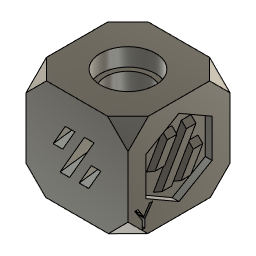
Voron_Design_Cube_v7 (Autodesk Fusion 360 design; units mm, degrees)
Autodesk Fusion 360 part; units mm, degrees
note: some values were not read from the file. Chosen so that the rebuilt part matches the saved one: which bodies a step acts on; the sign of a taper; which pieces of a blend or face edit are solid.
sketch "Sketch1" plane through (0, 0, 0) normal (1, 0, 0) x (0, 1, 0) in component "Voron_Design_Cube_v7"
  line L0 (15, -15) -> (-15, -15)
  line L1 (-15, -15) -> (-15, 15)
  line L2 (-15, 15) -> (15, 15)
  line L3 (15, 15) -> (15, -15)
  line L4 (15, -15) -> (-15, 15) construction
  line L5 (-15, -15) -> (15, 15) construction
  dimension "d4" = 30
  dimension "d5" = 30
  constraint horizontal L0
  constraint perpendicular L0 L1
  constraint parallel L0 L2
  constraint parallel L1 L3
  constraint coincident L4 origin
  constraint coincident L5 origin
  measures "d4" distance of L1.end L2.end
  measures "d5" distance of L0.end L1.end
extrude "Extrude1" add sketch "Sketch1" along normal mid plane 30 makes body 1 in component "Voron_Design_Cube_v7"
sketch "Sketch2" plane through (0, 0, 15) normal (0, 0, 1) x (-1, 0, 0) in component "Voron_Design_Cube_v7"
  line L0 (15, 15) -> (-15, 15)
  line L1 (-15, 15) -> (-15, -15)
  line L2 (-15, -15) -> (15, -15)
  line L3 (15, -15) -> (15, 15)
  circle A0 centre (0, 0) radius 8.1
  circle A1 centre (0, 0) radius 6.6
  dimension "d6" = 16.2
  dimension "d7" = 13.2
  constraint coincident A0.centre A1.centre
  measures "d6" diameter of A0
  measures "d7" diameter of A1
extrude "Extrude2" cut sketch "Sketch2" against normal through all contours A1 picked at (1.732843, 1.802463) bodies 1 in component "Voron_Design_Cube_v7"
extrude "Extrude3" cut sketch "Sketch2" against normal blind 5.2 contours A0 picked at (7.545271, -0.730307) bodies 1 in component "Voron_Design_Cube_v7"
sketch "Sketch3" plane through (0, 0, -15) normal (0, 0, -1) x (1, 0, 0) in component "Voron_Design_Cube_v7"
  circle A0 centre (0, 0) radius 6.6
  line L0 (-15, -15) -> (15, -15)
  line L1 (15, -15) -> (15, 15)
  line L2 (15, 15) -> (-15, 15)
  line L3 (-15, 15) -> (-15, -15)
  circle A1 centre (0, 0) radius 7.65
  dimension "d11" = 15.3
  constraint coincident A0.centre A1.centre
  measures "d11" diameter of A1
extrude "Extrude4" cut sketch "Sketch3" against normal blind 1.2 contours A0 | A1 picked at (1.732843, 1.802463) picked at (7.246947, -0.707951) bodies 1 in component "Voron_Design_Cube_v7"
sketch "Sketch4" plane through (0, 0, -13.8) normal (0, 0, -1) x (1, 0, 0) in component "Voron_Design_Cube_v7"
  circle A0 centre (0, 0) radius 6.6
  circle A1 centre (0, 0) radius 7.65
  circle A2 centre (0, 0) radius 7.625
  dimension "d14" = 15.25
  constraint concentric A0 A2
  measures "d14" diameter of A2
extrude "Extrude5" cut sketch "Sketch4" against normal through all draft -45 contours A0 | A1 A2 picked at (1.732843, 1.802463) picked at (7.246947, -0.707951) bodies 1 in component "Voron_Design_Cube_v7"
sketch "Sketch6" plane through (0, 0, 15) normal (0, 0, 1) x (-1, 0, 0) in component "Voron_Design_Cube_v7"
  circle A0 centre (0, 0) radius 8.1
  line L0 (15, 15) -> (-15, 15)
  line L1 (-15, 15) -> (-15, -15)
  line L2 (-15, -15) -> (15, -15)
  line L3 (15, -15) -> (15, 15)
  point P0 (9, -15)
  point P1 (15, -9)
  point P2 (15, 9)
  point P3 (9, 15)
  point P4 (-9, 15)
  point P5 (-15, 9)
  point P6 (-15, -9)
  point P7 (-9, -15)
  dimension "d20" = 6
  dimension "d21" = 6
  dimension "d23" = 360
  constraint coincident L2 P0
  constraint coincident L3 P1
  measures "d20" distance of L2.end P0
  measures "d21" distance of L2.end P1
sketch "Sketch7" plane through (0, 0, -15) normal (0, 0, -1) x (1, 0, 0) in component "Voron_Design_Cube_v7"
  circle A0 centre (0, 0) radius 7.65
  line L0 (-15, -15) -> (15, -15)
  line L1 (15, -15) -> (15, 15)
  line L2 (15, 15) -> (-15, 15)
  line L3 (-15, 15) -> (-15, -15)
  point P0 (-15, 9.040867)
  point P1 (-9, 15)
  point P2 (-15, -9)
  point P3 (-9.040867, -15)
  point P4 (9, -15)
  point P5 (15, -9.040867)
  point P6 (15, 9)
  point P7 (9.040867, 15)
  dimension "d25" = 360
  constraint coincident L2 P1
sketch "Sketch8" plane through (15, 0, 0) normal (1, 0, 0) x (0, 1, 0) in component "Voron_Design_Cube_v7"
  line L0 (15, 15) -> (-15, 15)
  line L1 (-15, 15) -> (-15, -15)
  line L2 (-15, -15) -> (15, -15)
  line L3 (15, -15) -> (15, 15)
  line L4 (0, 0) -> (0, 20) construction
  line L5 (0, 20) -> (0, 0) construction
  line L6 (0, 0) -> (20, 0) construction
  point P0 (-15, 9)
  point P1 (-15, 15)
  point P2 (15, 9)
  point P3 (-15, -9)
  point P4 (15, -9)
  dimension "d26" = 6
  constraint coincident L1 P0
  constraint coincident L4.start L5.end
  constraint vertical L4
  constraint parallel L4 L5
  constraint symmetric P0 L5 P2
  constraint perpendicular L5 L6
  constraint symmetric P0 L6 P3
  constraint symmetric P2 L6 P4
  measures "d26" distance of P0 P1
sketch "Sketch9" plane through (-15, 0, 0) normal (-1, 0, 0) x (0, -1, 0) in component "Voron_Design_Cube_v7"
  line L0 (15, 15) -> (-15, 15)
  line L1 (-15, 15) -> (-15, -15)
  line L2 (-15, -15) -> (15, -15)
  line L3 (15, -15) -> (15, 15)
  point P0 (-15, 9)
  point P1 (15, 9)
  point P2 (15, -9)
  point P3 (-15, -9)
ref_plane "WorkPlane1" through (-15, -9, 15) normal (0.57735, 0.57735, -0.57735) x (-0.707107, 0.707107, 0) in component "Voron_Design_Cube_v7"
ref_plane "WorkPlane2" through (9, -15, 15) normal (-0.57735, 0.57735, -0.57735) x (-0.707107, -0.707107, 0) in component "Voron_Design_Cube_v7"
ref_plane "WorkPlane3" through (15, 9, 15) normal (-0.57735, -0.57735, -0.57735) x (0.707107, -0.707107, 0) in component "Voron_Design_Cube_v7"
ref_plane "WorkPlane4" through (-9, 15, 15) normal (0.57735, -0.57735, -0.57735) x (0.707107, 0.707107, 0) in component "Voron_Design_Cube_v7"
ref_plane "WorkPlane5" through (-9.040867, 15, -15) normal (0.579981, -0.576031, 0.576031) x (0.704686, 0.709519, 0) in component "Voron_Design_Cube_v7"
ref_plane "WorkPlane6" through (-15, -9.040867, -15) normal (0.576031, 0.579981, 0.576031) x (-0.709519, 0.704686, 0) in component "Voron_Design_Cube_v7"
ref_plane "WorkPlane7" through (9.040867, -15, -15) normal (-0.579981, 0.576031, 0.576031) x (-0.704686, -0.709519, 0) in component "Voron_Design_Cube_v7"
ref_plane "WorkPlane8" through (15, 9.040867, -15) normal (-0.576031, -0.579981, 0.576031) x (0.709519, -0.704686, 0) in component "Voron_Design_Cube_v7"
split "Split1" by plane through (9, -15, 15) normal (-0.57735, 0.57735, -0.57735) bodies 1 makes body 2 at (6.567203, -0.657148, -5.25) in component "Voron_Design_Cube_v7"
delete_body "RemoveBody1" bodies 1 in component "Voron_Design_Cube_v7"
split "Split2" by plane through (15, 9, 15) normal (-0.57735, -0.57735, -0.57735) bodies 2 makes body 3 at (6.567203, -0.657148, -5.25) in component "Voron_Design_Cube_v7"
delete_body "RemoveBody2" bodies 2 in component "Voron_Design_Cube_v7"
split "Split3" by plane through (-9, 15, 15) normal (0.57735, -0.57735, -0.57735) bodies 3 makes body 4 at (6.567203, -0.657148, -5.25) in component "Voron_Design_Cube_v7"
delete_body "RemoveBody3" bodies 3 in component "Voron_Design_Cube_v7"
split "Split4" by plane through (-15, -9, 15) normal (0.57735, 0.57735, -0.57735) bodies 4 makes body 5 at (6.567203, -0.657148, -5.25) in component "Voron_Design_Cube_v7"
delete_body "RemoveBody4" bodies 4 in component "Voron_Design_Cube_v7"
split "Split5" by plane through (-15, -9.040867, -15) normal (0.576031, 0.579981, 0.576031) bodies 5 makes body 6 at (6.567203, -0.657148, -5.25) in component "Voron_Design_Cube_v7"
delete_body "RemoveBody5" bodies 5 in component "Voron_Design_Cube_v7"
split "Split6" by plane through (9.040867, -15, -15) normal (-0.579981, 0.576031, 0.576031) bodies 6 makes body 7 at (6.567203, -0.657148, -5.25) in component "Voron_Design_Cube_v7"
delete_body "RemoveBody6" bodies 6 in component "Voron_Design_Cube_v7"
split "Split7" by plane through (15, 9.040867, -15) normal (-0.576031, -0.579981, 0.576031) bodies 7 makes body 8 at (6.567203, -0.657148, -5.25) in component "Voron_Design_Cube_v7"
delete_body "RemoveBody7" bodies 7 in component "Voron_Design_Cube_v7"
split "Split8" by plane through (-9.040867, 15, -15) normal (0.579981, -0.576031, 0.576031) bodies 8 makes body 9 at (6.567203, -0.657148, -5.25) in component "Voron_Design_Cube_v7"
delete_body "RemoveBody8" bodies 8 in component "Voron_Design_Cube_v7"
sketch "Sketch10" plane through (0, 15, 0) normal (0, 1, 0) x (-1, 0, 0) in component "Voron_Design_Cube_v7"
  line L0 (9.040866, -15) -> (15, -9)
  line L1 (15, -9) -> (15, 9)
  line L2 (15, 9) -> (9, 15)
  line L3 (9, 15) -> (-9, 15)
  line L4 (-9, 15) -> (-15, 9)
  line L5 (-15, 9) -> (-15, -9)
  line L6 (-15, -9) -> (-9, -15)
  line L7 (-9, -15) -> (9.040866, -15)
  line L8 (-13, -13) -> (-7.5, -13) construction
  line L9 (-7.5, -13) -> (-7.5, -7) construction
  line L10 (-7.5, -7) -> (-13, -7) construction
  line L11 (-13, -7) -> (-13, -13) construction
  dimension "d27" = 5.7
  dimension "d30" = 13
  dimension "d31" = 13
  text T0 "X" font "Arial" height 5.7 align left bottom in box 5.5 x 6 at (-13, -13) x (1, 0) y (0, 1) spacing 1
  measures "d30" distance of origin
  measures "d31" distance of origin
extrude "Extrude6" cut sketch "Sketch10" against normal blind 2 text T0 bodies 9 in component "Voron_Design_Cube_v7"
sketch "Sketch11" plane through (15, 0, 0) normal (1, 0, 0) x (0, 1, 0) in component "Voron_Design_Cube_v7"
  line L0 (9.040867, -15) -> (15, -9)
  line L1 (15, -9) -> (15, 9)
  line L2 (15, 9) -> (9, 15)
  line L3 (9, 15) -> (-9, 15)
  line L4 (-9, 15) -> (-15, 9)
  line L5 (-15, 9) -> (-15, -9)
  line L6 (-15, -9) -> (-9, -15)
  line L7 (-9, -15) -> (9.040867, -15)
  line L8 (-13, -13) -> (-5.617602, -13) construction
  line L9 (-5.617602, -13) -> (-5.617602, -5.858994) construction
  line L10 (-5.617602, -5.858994) -> (-13, -5.858994) construction
  line L11 (-13, -5.858994) -> (-13, -13) construction
  dimension "d32" = 5.7
  dimension "d33" = 13
  dimension "d34" = 13
  text T0 "Y" font "Arial" height 5.7 align left bottom in box 7.382398 x 7.141006 at (-13, -13) x (1, 0) y (0, 1) spacing 1
  constraint horizontal L8
  measures "d33" distance of origin
  measures "d34" distance of origin
extrude "Extrude7" cut sketch "Sketch11" against normal blind 2 text T0 bodies 9 in component "Voron_Design_Cube_v7"
sketch "Sketch12" plane through (15, 0, 0) normal (1, 0, 0) x (0, 1, 0) in component "Voron_Design_Cube_v7"
  line L0 (-9.73799, 5.622396) -> (0, 11.244792)
  line L1 (0, 11.244792) -> (9.73799, 5.622396)
  line L2 (9.73799, 5.622396) -> (9.73799, -5.622396)
  line L3 (9.73799, -5.622396) -> (0, -11.244792)
  line L4 (0, -11.244792) -> (-9.73799, -5.622396)
  line L5 (-9.73799, -5.622396) -> (-9.73799, 5.622396)
  line L6 (-7.01675, 0) -> (-3.440906, 6.207125)
  line L7 (-3.440906, 6.207125) -> (-0.629708, 6.207125)
  line L8 (-0.629708, 6.207125) -> (-4.205552, 0)
  line L9 (-4.205552, 0) -> (-7.01675, 0)
  line L10 (2.18149, 6.207125) -> (4.992688, 6.207125)
  line L11 (4.992688, 6.207125) -> (-2.18149, -6.207125)
  line L12 (-2.18149, -6.207125) -> (-4.992688, -6.207125)
  line L13 (-4.992688, -6.207125) -> (2.18149, 6.207125)
  line L14 (4.205552, 0) -> (7.01675, 0)
  line L15 (7.01675, 0) -> (3.440906, -6.207125)
  line L16 (3.440906, -6.207125) -> (0.629708, -6.207125)
  line L17 (0.629708, -6.207125) -> (4.205552, 0)
extrude "Extrude8" cut sketch "Sketch12" against normal blind 2 bodies 9 in component "Voron_Design_Cube_v7"
draft "Draft1" angle 25 neutral plane through (15, 0, 0) pull (1, 0, 0) 6 faces at (14.333333, -2.50384, 6.207125) (14.333333, 3.118556, 6.207125) (14.333333, 5.142618, 0) (14.333333, -3.118556, -6.207125) (14.333333, 2.50384, -6.207125) (14.333333, -5.142618, 0) on bodies 9 in component "Voron_Design_Cube_v7"
sketch "Sketch13" plane through (-15, 0, 0) normal (-1, 0, 0) x (0, -1, 0) in component "Voron_Design_Cube_v7"
  line L0 (-15, -9) -> (-9, -15)
  line L1 (-9, -15) -> (9.040867, -15)
  line L2 (9.040867, -15) -> (15, -9)
  line L3 (15, -9) -> (15, 9)
  line L4 (15, 9) -> (9, 15)
  line L5 (9, 15) -> (-9, 15)
  line L6 (-9, 15) -> (-15, 9)
  line L7 (-15, 9) -> (-15, -9)
  line L8 (-9.73799, 5.622396) -> (0, 11.244792)
  line L9 (0, 11.244792) -> (9.73799, 5.622396)
  line L10 (9.73799, 5.622396) -> (9.73799, -5.622396)
  line L11 (9.73799, -5.622396) -> (0, -11.244792)
  line L12 (0, -11.244792) -> (-9.73799, -5.622396)
  line L13 (-9.73799, -5.622396) -> (-9.73799, 5.622396)
  line L14 (-7.01675, 0) -> (-3.440906, 6.207125)
  line L15 (-3.440906, 6.207125) -> (-0.629708, 6.207125)
  line L16 (-0.629708, 6.207125) -> (-4.205552, 0)
  line L17 (-4.205552, 0) -> (-7.01675, 0)
  line L18 (2.18149, 6.207125) -> (4.992688, 6.207125)
  line L19 (4.992688, 6.207125) -> (-2.18149, -6.207125)
  line L20 (-2.18149, -6.207125) -> (-4.992688, -6.207125)
  line L21 (-4.992688, -6.207125) -> (2.18149, 6.207125)
  line L22 (4.205552, 0) -> (7.01675, 0)
  line L23 (7.01675, 0) -> (3.440906, -6.207125)
  line L24 (3.440906, -6.207125) -> (0.629708, -6.207125)
  line L25 (0.629708, -6.207125) -> (4.205552, 0)
extrude "Extrude9" cut sketch "Sketch13" against normal blind 2 contours L8 L9 L10 L11 L12 L13 picked at (-6.731882, 3.943174) bodies 9 in component "Voron_Design_Cube_v7"
draft "Draft2" angle 25 neutral plane through (-15, 0, 0) pull (-1, 0, 0) 5 faces at (-14.333333, 2.50384, 6.207125) (-14.333333, -3.118556, 6.207125) (-14.333333, -5.142618, 0) (-14.333333, -2.50384, -6.207125) (-14.333333, 3.118556, -6.207125) on bodies 9 in component "Voron_Design_Cube_v7"
sketch "Sketch14" plane through (0, 15, 0) normal (0, 1, 0) x (-1, 0, 0) in component "Voron_Design_Cube_v7"
  line L0 (-10.663234, -11.013165) -> (-11.636027, -12.363973)
  line L1 (-11.636027, -12.363973) -> (-9, -15)
  line L2 (-9, -15) -> (9.040866, -15)
  line L3 (9.040866, -15) -> (15, -9)
  line L4 (15, -9) -> (15, 9)
  line L5 (15, 9) -> (9, 15)
  line L6 (9, 15) -> (-9, 15)
  line L7 (-9, 15) -> (-15, 9)
  line L8 (-15, 9) -> (-15, -9)
  line L9 (-15, -9) -> (-12.148009, -11.851991)
  line L10 (-12.148009, -11.851991) -> (-10.79543, -10.029468)
  line L11 (-10.79543, -10.029468) -> (-12.739495, -7.3)
  line L12 (-12.739495, -7.3) -> (-11.841337, -7.3)
  line L13 (-11.841337, -7.3) -> (-10.807095, -8.761938)
  spline S0 degree 3 poles (-10.807095, -8.761938) (-10.713074, -8.894778) (-10.551797, -9.122645) (-10.408185, -9.361989) (-10.348295, -9.461801) knots 0 0 0 0 0.04880071 0.08371009 0.08371009 0.08371009 0.08371009
  spline S1 degree 3 poles (-10.348295, -9.461801) (-10.280285, -9.354929) (-10.138691, -9.132428) (-9.979829, -8.921894) (-9.897272, -8.812483) knots 0 0 0 0 0.03798709 0.07908704 0.07908704 0.07908704 0.07908704
  line L14 (-9.897272, -8.812483) -> (-8.750273, -7.3)
  line L15 (-8.750273, -7.3) -> (-7.929878, -7.3)
  line L16 (-7.929878, -7.3) -> (-9.932265, -9.986699)
  line L17 (-9.932265, -9.986699) -> (-7.774352, -13)
  line L18 (-7.774352, -13) -> (-8.707504, -13)
  line L19 (-8.707504, -13) -> (-10.142224, -10.966508)
  spline S2 degree 3 poles (-10.142224, -10.966508) (-10.183392, -10.905818) (-10.268563, -10.780259) (-10.349334, -10.651825) (-10.391065, -10.585471) knots 0 0 0 0 0.02199887 0.04551245 0.04551245 0.04551245 0.04551245
  spline S3 degree 3 poles (-10.391065, -10.585471) (-10.444812, -10.673394) (-10.532967, -10.817603) (-10.626663, -10.958264) (-10.663234, -11.013165) knots 0 0 0 0 0.03091064 0.05069909 0.05069909 0.05069909 0.05069909
  line L20 (-9.73799, 5.622396) -> (0, 11.244792)
  line L21 (0, 11.244792) -> (9.73799, 5.622396)
  line L22 (9.73799, 5.622396) -> (9.73799, -5.622396)
  line L23 (9.73799, -5.622396) -> (0, -11.244792)
  line L24 (0, -11.244792) -> (-9.73799, -5.622396)
  line L25 (-9.73799, -5.622396) -> (-9.73799, 5.622396)
  line L26 (-7.01675, 0) -> (-3.440906, 6.207125)
  line L27 (-3.440906, 6.207125) -> (-0.629708, 6.207125)
  line L28 (-0.629708, 6.207125) -> (-4.205552, 0)
  line L29 (-4.205552, 0) -> (-7.01675, 0)
  line L30 (2.18149, 6.207125) -> (4.992688, 6.207125)
  line L31 (4.992688, 6.207125) -> (-2.18149, -6.207125)
  line L32 (-2.18149, -6.207125) -> (-4.992688, -6.207125)
  line L33 (-4.992688, -6.207125) -> (2.18149, 6.207125)
  line L34 (4.205552, 0) -> (7.01675, 0)
  line L35 (7.01675, 0) -> (3.440906, -6.207125)
  line L36 (3.440906, -6.207125) -> (0.629708, -6.207125)
  line L37 (0.629708, -6.207125) -> (4.205552, 0)
sketch "Sketch15" plane through (0, -15, 0) normal (0, -1, 0) x (1, 0, 0) in component "Voron_Design_Cube_v7"
  line L0 (9.040866, -15) -> (15, -9)
  line L1 (15, -9) -> (15, 9)
  line L2 (15, 9) -> (9, 15)
  line L3 (9, 15) -> (-9, 15)
  line L4 (-9, 15) -> (-15, 9)
  line L5 (-15, 9) -> (-15, -9)
  line L6 (-15, -9) -> (-9, -15)
  line L7 (-9, -15) -> (9.040866, -15)
  line L8 (-9.73799, 5.622396) -> (0, 11.244792)
  line L9 (0, 11.244792) -> (9.73799, 5.622396)
  line L10 (9.73799, 5.622396) -> (9.73799, -5.622396)
  line L11 (9.73799, -5.622396) -> (0, -11.244792)
  line L12 (0, -11.244792) -> (-9.73799, -5.622396)
  line L13 (-9.73799, -5.622396) -> (-9.73799, 5.622396)
  line L14 (-7.01675, 0) -> (-3.440906, 6.207125)
  line L15 (-3.440906, 6.207125) -> (-0.629708, 6.207125)
  line L16 (-0.629708, 6.207125) -> (-4.205552, 0)
  line L17 (-4.205552, 0) -> (-7.01675, 0)
  line L18 (2.18149, 6.207125) -> (4.992688, 6.207125)
  line L19 (4.992688, 6.207125) -> (-2.18149, -6.207125)
  line L20 (-2.18149, -6.207125) -> (-4.992688, -6.207125)
  line L21 (-4.992688, -6.207125) -> (2.18149, 6.207125)
  line L22 (4.205552, 0) -> (7.01675, 0)
  line L23 (7.01675, 0) -> (3.440906, -6.207125)
  line L24 (3.440906, -6.207125) -> (0.629708, -6.207125)
  line L25 (0.629708, -6.207125) -> (4.205552, 0)
extrude "Extrude1'" add sketch "Sketch14" against normal blind 30 separate body contours L26 L27 L28 L29 | L30 L31 L32 L33 | L34 L35 L36 L37 picked at (-4.887736, 2.069042) picked at (-1.664229, -2.069042) picked at (2.758722, -4.138083) makes body 10 at (5.824802, 5, 2.069042) makes body 11 at (-2.601295, 5, 2.069042) makes body 12 at (-5.824802, 5, -2.069042) in component "cutting tool 1"
draft "Draft1'" angle -20.5 neutral plane through (0, 15, 0) pull (0, 1, 0) 6 faces at (1.566774, 5, 6.207125) (6.079684, 5, 0) (-3.118556, -5, 6.207125) (3.118556, -5, -6.207125) (-1.566774, 5, -6.207125) (-6.079684, 5, 0) on bodies 10 11 12 in component "cutting tool 1"
combine "Combine1" operation cut target body 9 tool bodies 10 11 12 in component "Voron_Design_Cube_v7"
extrude "Extrude1''" add sketch "Sketch15" against normal blind 30 separate body contours L14 L15 L16 L17 | L18 L19 L20 L21 | L22 L23 L24 L25 picked at (-4.887736, 2.069042) picked at (-1.664229, -2.069042) picked at (2.758722, -4.138083) makes body 13 at (-5.824802, -5, 2.069042) makes body 14 at (2.601295, -5, 2.069042) makes body 15 at (5.824802, -5, -2.069042) in component "cutting tool 2"
draft "Draft1''" angle -20.5 neutral plane through (0, -15, 0) pull (0, -1, 0) 6 faces at (-1.566774, -5, 6.207125) (3.118556, 5, 6.207125) (6.079684, -5, 0) (-3.118556, 5, -6.207125) (1.566774, -5, -6.207125) (-6.079684, -5, 0) on bodies 13 14 15 in component "cutting tool 2"
combine "Combine2" operation cut target body 9 tool bodies 13 15 14 in component "Voron_Design_Cube_v7"
sketch "Sketch16" plane through (0, 0, 0) normal (0, 0, 1) x (1, 0, 0) in component "Voron_Design_Cube_v7"
  circle A0 centre (0, 0) radius 6.6
  line L0 (-5.531727, 3.6) -> (5.531727, 3.6)
  line L1 (5.531727, -3.6) -> (-5.531727, -3.6)
  line L2 (0, 0) -> (17.5, 0) construction
  dimension "d54" = 3.6
  constraint horizontal L0
  constraint parallel L0 L1
  constraint coincident A0.centre L2.start
  constraint horizontal L2
  constraint symmetric L0 L1 L2
  measures "d54" distance of A0.centre L0
extrude "Extrude10" add sketch "Sketch16" along normal mid plane 0.8 contours A0 L0 L1 picked at (1.843909, 0.567574) bodies 9 in component "Voron_Design_Cube_v7"
chamfer "Chamfer1" distance 0.2 angle 45 9 edges at (12, 12.020433, -15) (-0.020433, 15, -15) (-12.020433, 12, -15) (-15, -0.020433, -15) (-12, -12.020433, -15) (0.020433, -15, -15) (12.020433, -12, -15) (15, 0.020433, -15) (-7.132304, -2.766358, -15) on bodies 9 in component "Voron_Design_Cube_v7"
component "Voron_Design_Cube_v7" placed x (1, 0, 0) y (0, 1, 0) z (0, 0, 1) at (0, 0, 0)
component "cutting tool 1" placed x (1, 0, 0) y (0, 1, 0) z (0, 0, 1) at (0, 0, 0) in component "Voron_Design_Cube_v7"
component "cutting tool 2" placed x (1, 0, 0) y (0, 1, 0) z (0, 0, 1) at (0, 0, 0) in component "Voron_Design_Cube_v7"
equation "d1 = size"
equation "size = 30 mm"
equation "d4 = size"
equation "d5 = size"
equation "d20 = size * 0.2"
equation "d21 = size * 0.2"
equation "d26 = size * 0.2"
equation "d27 = size / 30 * 5.7"
equation "d30 = size / 30 * 13"
equation "d31 = size / 30 * 13"
equation "d32 = size / 30 * 5.70"
equation "d33 = size / 30 * 13"
equation "d34 = size / 30 * 13"
equation "d45 = -size"
equation "d49 = -size"
